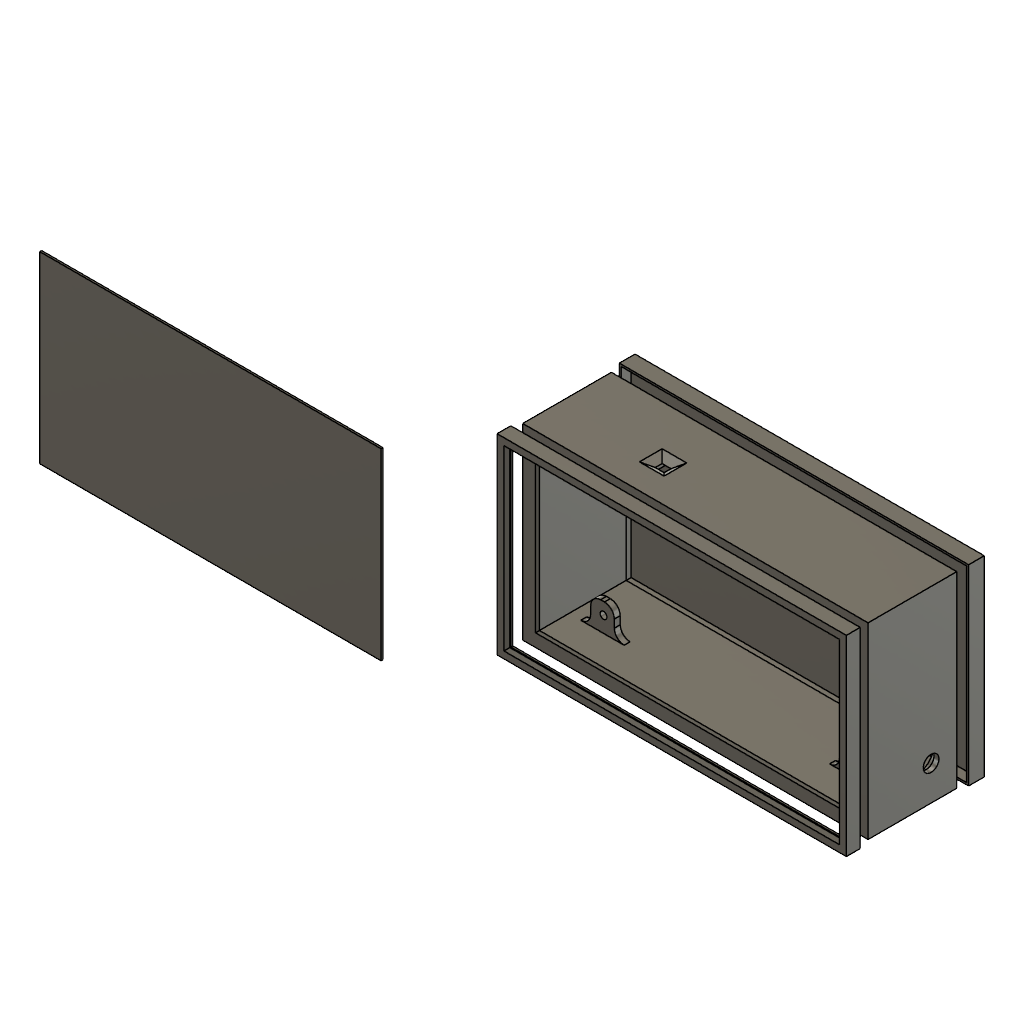
Bedroom Clock (Autodesk Fusion 360 design; units mm, degrees)
Autodesk Fusion 360 part; units mm, degrees
sketch "Sketch1" plane through (0, 0, 0) normal (0, 0, 1) x (1, 0, 0)
  line L0 (80.1, -40.1) -> (-80.1, -40.1)
  line L1 (-80.1, -40.1) -> (-80.1, 40.1)
  line L2 (-80.1, 40.1) -> (80.1, 40.1)
  line L3 (80.1, 40.1) -> (80.1, -40.1)
  line L4 (80.1, -40.1) -> (-80.1, 40.1) construction
  line L5 (-80.1, -40.1) -> (80.1, 40.1) construction
  line L6 (87.6, -47.6) -> (-87.6, -47.6)
  line L7 (-87.6, -47.6) -> (-87.6, 47.6)
  line L8 (-87.6, 47.6) -> (87.6, 47.6)
  line L9 (87.6, 47.6) -> (87.6, -47.6)
  dimension "d1" = 160.2
  dimension "d2" = 80.2
  dimension "d3" = -7.5
  constraint horizontal L0
  constraint perpendicular L0 L1
  constraint parallel L0 L2
  constraint parallel L1 L3
  constraint coincident L4 origin
  constraint coincident L5 origin
  measures "d1" distance of L1.end L2.end
  measures "d2" distance of L0.end L1.end
extrude "Extrude1" add sketch "Sketch1" along normal blind 30 makes body 1
sketch "Sketch2" plane through (0, -40.1, 0) normal (0, 1, 0) x (-1, 0, 0)
  line L0 (-80.1, 0) -> (80.1, 0)
  line L1 (80.1, 0) -> (80.1, 30)
  line L2 (80.1, 30) -> (-80.1, 30)
  line L3 (-80.1, 30) -> (-80.1, 0)
  line L4 (69.1, 11) -> (57.1, 11)
  line L5 (57.1, 11) -> (57.1, 14)
  line L6 (57.1, 14) -> (69.1, 14)
  line L7 (69.1, 14) -> (69.1, 11)
  line L8 (-57.1, 11) -> (-69.1, 11)
  line L9 (-69.1, 11) -> (-69.1, 14)
  line L10 (-69.1, 14) -> (-57.1, 14)
  line L11 (-57.1, 14) -> (-57.1, 11)
  dimension "d6" = 12
  dimension "d7" = 11
  dimension "d8" = 16
  dimension "d9" = 12
  dimension "d10" = 3
  dimension "d11" = 16
  dimension "d12" = 11
  constraint horizontal L4
  constraint vertical L5
  constraint horizontal L6
  constraint vertical L7
  constraint horizontal L8
  constraint vertical L9
  constraint horizontal L10
  constraint vertical L11
  measures "d6" distance of L4.start L4.end
  measures "d7" distance of L1 L7
  measures "d8" distance of L2 L6
  measures "d9" distance of L8.start L8.end
  measures "d10" distance of L8.start L10.end
  measures "d11" distance of L2 L10
  measures "d12" distance of L3 L9
extrude "Extrude2" add sketch "Sketch2" along normal blind 14 contours L4 L5 L6 L7 | L8 L9 L10 L11 bodies 1
mirror "Mirror1" about plane through (0, 0, 0) normal (0, 1, 0) of "Extrude2"
fillet "Fillet2" radius 5 16 edges at (-57.1, -40.1, 12.5) (-57.1, -26.1, 12.5) (-69.1, -26.1, 12.5) (-69.1, -40.1, 12.5) (57.1, -40.1, 12.5) (57.1, -26.1, 12.5) (69.1, -26.1, 12.5) (69.1, -40.1, 12.5) (-57.1, 40.1, 12.5) (-57.1, 26.1, 12.5) (-69.1, 26.1, 12.5) (-69.1, 40.1, 12.5) (57.1, 40.1, 12.5) (57.1, 26.1, 12.5) (69.1, 26.1, 12.5) (69.1, 40.1, 12.5) on bodies 1
sketch "Sketch4" plane through (0, 0, 14) normal (0, 0, 1) x (1, 0, 0)
  arc A0 (-64.1, -26.1) -> (-69.1, -31.1) centre (-64.1, -31.1) ccw
  line L0 (-69.1, -31.1) -> (-69.1, -35.1)
  arc A1 (-74.1, -40.1) -> (-69.1, -35.1) centre (-74.1, -35.1) ccw
  line L1 (-74.1, -40.1) -> (-52.1, -40.1)
  arc A2 (-57.1, -35.1) -> (-52.1, -40.1) centre (-52.1, -35.1) ccw
  line L2 (-57.1, -35.1) -> (-57.1, -31.1)
  arc A3 (-57.1, -31.1) -> (-62.1, -26.1) centre (-62.1, -31.1) ccw
  line L3 (-62.1, -26.1) -> (-64.1, -26.1)
  circle A4 centre (-62.57, -32.17) radius 1.75
  line L4 (-74.1, -40.1) -> (-52.1, -40.1)
  circle A5 centre (62.57, -32.17) radius 1.75
  line L5 (74.1, -40.1) -> (52.1, -40.1)
  circle A6 centre (62.57, 32.17) radius 1.75
  line L6 (52.1, 40.1) -> (74.1, 40.1)
  circle A7 centre (-62.57, 32.17) radius 1.75
  line L7 (-74.1, 40.1) -> (-52.1, 40.1)
  point P0 (-80.1, -40.1)
  point P1 (80.1, -40.1)
  point P2 (80.1, 40.1)
  point P3 (-80.1, 40.1)
  dimension "d28" = 3.5
  dimension "d29" = 7.93
  dimension "d30" = 17.53
  dimension "d31" = 3.5
  dimension "d32" = 7.93
  dimension "d33" = 17.53
  dimension "d34" = 3.5
  dimension "d35" = 7.93
  dimension "d36" = 17.53
  dimension "d37" = 3.5
  dimension "d38" = 7.93
  dimension "d39" = 17.53
  measures "d28" diameter of A4
  measures "d29" distance of A4.centre L4
  measures "d30" horizontal distance of A4.centre P0
  measures "d31" diameter of A5
  measures "d32" distance of A5.centre L5
  measures "d33" horizontal distance of A5.centre P1
  measures "d34" diameter of A6
  measures "d35" distance of A6.centre L6
  measures "d36" horizontal distance of A6.centre P2
  measures "d37" diameter of A7
  measures "d38" distance of A7.centre L7
  measures "d39" horizontal distance of A7.centre P3
extrude "Extrude4" cut sketch "Sketch4" against normal blind 3 contours A4 | A5 | A6 | A7 bodies 1
chamfer "Chamfer1" distance 1 angle 45 4 edges at (-80.1, 0, 30) (0, -40.1, 30) (0, 40.1, 30) (80.1, 0, 30) tangent chain off on bodies 1
ref_plane "WorkPlane1" through (0, 0, 10) normal (0, 0, 1) x (1, 0, 0) in component "ESP32 Mount"
sketch "Sketch1 (2)" plane through (0, 0, 10) normal (0, 0, 1) x (1, 0, 0) in component "ESP32 Mount"
  line L0 (62, -36.7675) -> (-62, -36.7675)
  line L1 (-70, -28.7675) -> (-70, 28.7675)
  line L2 (-62, 36.7675) -> (62, 36.7675)
  line L3 (70, 28.7675) -> (70, -28.7675)
  line L4 (5, -9.7675) -> (-14, -9.7675)
  line L5 (-14, -9.7675) -> (-14, 10.2325)
  line L6 (-14, 10.2325) -> (5, 10.2325)
  line L7 (5, 10.2325) -> (5, -9.7675)
  circle A0 centre (-62.57, 32.17) radius 1.75
  circle A1 centre (-62.57, -32.17) radius 1.75
  circle A2 centre (62.57, -32.17) radius 1.75
  circle A3 centre (62.57, 32.17) radius 1.75
  line L8 (-46.57, 15.83) -> (-31.57, 15.83)
  line L9 (-31.57, 15.83) -> (-31.57, -17.17)
  line L10 (-31.57, -17.17) -> (-46.57, -17.17)
  line L11 (-46.57, -17.17) -> (-46.57, 15.83)
  circle A4 centre (18.7, 12.17) radius 1.5
  circle A5 centre (59, 12.17) radius 1.5
  circle A6 centre (18.7, -7.13) radius 1.5
  circle A7 centre (59, -7.13) radius 1.5
  arc A8 (-62, 36.7675) -> (-70, 28.7675) centre (-62, 28.7675) ccw
  arc A9 (-70, -28.7675) -> (-62, -36.7675) centre (-62, -28.7675) ccw
  arc A10 (62, -36.7675) -> (70, -28.7675) centre (62, -28.7675) ccw
  arc A11 (70, 28.7675) -> (62, 36.7675) centre (62, 28.7675) ccw
  dimension "d45" = 65
  dimension "d46" = 27
  dimension "d48" = 15
  dimension "d49" = 33
  dimension "d50" = 15
  dimension "d51" = 16
  dimension "d52" = 3
  dimension "d53" = 3
  dimension "d54" = 3
  dimension "d55" = 3
  dimension "d56" = 19.3
  dimension "d57" = 19.3
  dimension "d58" = 40.3
  dimension "d59" = 40.3
  dimension "d60" = 11
  dimension "d61" = 11
  dimension "d62" = 20
  dimension "d63" = 20
  dimension "d64" = 8
  dimension "d67" = 19
  dimension "d68" = 140
  dimension "d69" = 20
  constraint horizontal L0
  constraint perpendicular L0 L1
  constraint parallel L0 L2
  constraint parallel L1 L3
  constraint horizontal L4
  constraint perpendicular L4 L5
  constraint parallel L4 L6
  constraint parallel L5 L7
  constraint horizontal L8
  constraint vertical L9
  constraint horizontal L10
  constraint vertical L11
  constraint tangent L2 A8
  constraint tangent L1 A8
  constraint tangent L0 A9
  constraint tangent L1 A9
  constraint equal A8 A9
  constraint tangent L0 A10
  constraint tangent L3 A10
  constraint equal A8 A10
  constraint tangent L3 A11
  constraint tangent L2 A11
  constraint equal A8 A11
  measures "d45" distance of L3 L7
  measures "d46" distance of L0 L4
  measures "d48" distance of L8.start L8.end
  measures "d49" distance of L8.start L10.end
  measures "d50" distance of A1.centre L10
  measures "d51" distance of A0.centre L11
  measures "d52" diameter of A4
  measures "d53" diameter of A5
  measures "d54" diameter of A6
  measures "d55" diameter of A7
  measures "d56" vertical distance of A5.centre A7.centre
  measures "d57" vertical distance of A4.centre A6.centre
  measures "d58" horizontal distance of A6.centre A7.centre
  measures "d59" horizontal distance of A4.centre A5.centre
  measures "d60" distance of L3 A7.centre
  measures "d61" distance of L3 A5.centre
  measures "d62" vertical distance of A3.centre A5.centre
  measures "d63" vertical distance of A3.centre A4.centre
  measures "d64" radius of A8
  measures "d67" distance of L5 L7
  measures "d68" distance of L1 L3
  measures "d69" distance of L4 L6
extrude "Extrude1'" add sketch "Sketch1 (2)" along normal blind 3 separate body makes body 2 in component "ESP32 Mount"
move_body "Move1" bodies 2 to x (1, 0, 0) y (0, 1, 0) z (0, 0, 1) at (0, 0, 65) in component "ESP32 Mount"
copy_body "Body->Comp1" bodies 1 removing the originals makes body 3 in component "Display Frame"
sketch "Sketch1 (3)" plane through (0, 40.1, 0) normal (0, -1, 0) x (1, 0, 0) in component "Display Frame"
  line L0 (80.1, 29) -> (-80.1, 29)
  line L1 (-80.1, 29) -> (-80.1, 0)
  line L2 (-80.1, 0) -> (80.1, 0)
  line L3 (80.1, 0) -> (80.1, 29)
  line L4 (74.1, 11) -> (52.1, 11)
  line L5 (52.1, 11) -> (52.1, 14)
  line L6 (52.1, 14) -> (74.1, 14)
  line L7 (74.1, 14) -> (74.1, 11)
  line L8 (-74.1, 14) -> (-52.1, 14)
  line L9 (-52.1, 14) -> (-52.1, 11)
  line L10 (-52.1, 11) -> (-74.1, 11)
  line L11 (-74.1, 11) -> (-74.1, 14)
  line L12 (-28.5, 0) -> (-42.1, 0)
  line L13 (-42.1, 0) -> (-42.1, 18.5)
  line L14 (-42.1, 18.5) -> (-28.5, 18.5)
  line L15 (-28.5, 18.5) -> (-28.5, 0)
  line L16 (-32.6, 9.75) -> (-37.1, 9.75)
  line L17 (-37.1, 9.75) -> (-37.1, 13.25)
  line L18 (-37.1, 13.25) -> (-32.6, 13.25)
  line L19 (-32.6, 13.25) -> (-32.6, 9.75)
  dimension "d70" = 38
  dimension "d71" = 13.6
  dimension "d72" = 18.5
  dimension "d73" = 4.5
  dimension "d74" = 3.5
  dimension "d75" = 5
  dimension "d76" = 5.25
  constraint horizontal L12
  constraint vertical L13
  constraint horizontal L14
  constraint vertical L15
  constraint coincident L2 L12.start
  constraint horizontal L16
  constraint vertical L17
  constraint horizontal L18
  constraint vertical L19
  measures "d70" distance of L1 L13
  measures "d71" distance of L13 L15
  measures "d72" distance of L12 L14
  measures "d73" distance of L16.start L16.end
  measures "d74" distance of L16.start L18.end
  measures "d75" distance of L13 L17
  measures "d76" distance of L14 L18
extrude "Extrude1''" cut sketch "Sketch1 (3)" against normal blind 5 contours L2 L12 L13 L14 L15 bodies 3 in component "Display Frame"
extrude "Extrude2'" cut 1 faces at (-34.1, 40.1, 12.0833) along direction (0, 1, 0) blind 7.5 on bodies 3 bodies 3 in component "Display Frame"
chamfer "Chamfer1'" distance 4 distance2 2.5 4 edges at (-34.85, 47.6, 13.25) (-32.6, 47.6, 11.5) (-34.85, 47.6, 9.75) (-37.1, 47.6, 11.5) measured on face at (47.5333, 47.6, 14.4167) measured on face at (47.5333, 47.6, 14.4167) measured on face at (47.5333, 47.6, 14.4167) measured on face at (47.5333, 47.6, 14.4167) tangent chain off on bodies 3 in component "Display Frame"
sketch "Sketch2 (2)" plane through (-28.5, 0, 0) normal (-1, 0, 0) x (0, 0, 1) in component "Display Frame"
  line L0 (0, 40.1) -> (18.5, 40.1)
  line L1 (18.5, 40.1) -> (18.5, 45.1)
  line L2 (18.5, 45.1) -> (0, 45.1)
  line L3 (0, 45.1) -> (0, 40.1)
  line L4 (18.5, 42.5) -> (4, 42.5)
  line L5 (4, 42.5) -> (4, 40.5)
  line L6 (4, 40.5) -> (18.5, 40.5)
  line L7 (18.5, 40.5) -> (18.5, 42.5)
  dimension "d82" = 14.5
  dimension "d83" = 2
  dimension "d84" = 2.6
  constraint horizontal L4
  constraint vertical L5
  constraint horizontal L6
  constraint vertical L7
  measures "d82" distance of L4.start L4.end
  measures "d83" distance of L4.start L6.end
  measures "d84" distance of L2 L4
extrude "Extrude3" add sketch "Sketch2 (2)" along normal blind 2 contours L1 L4 L5 L6 L7 bodies 3 in component "Display Frame"
chamfer "Chamfer2" distance 2 distance2 1 1 edges at (-29.5, 42.5, 4) measured on face at (-29.1667, 42.5, 13.6667) tangent chain off on bodies 3 in component "Display Frame"
sketch "Sketch3" plane through (-42.1, 0, 0) normal (1, 0, 0) x (0, 0, -1) in component "Display Frame"
  line L0 (-18.5, 40.1) -> (0, 40.1)
  line L1 (0, 40.1) -> (0, 45.1)
  line L2 (0, 45.1) -> (-18.5, 45.1)
  line L3 (-18.5, 45.1) -> (-18.5, 40.1)
  line L4 (-18.5, 42.5) -> (-4, 42.5)
  line L5 (-4, 42.5) -> (-4, 40.5)
  line L6 (-4, 40.5) -> (-18.5, 40.5)
  line L7 (-18.5, 40.5) -> (-18.5, 42.5)
  dimension "d89" = 14.5
  dimension "d90" = 2
  dimension "d91" = 2.6
  constraint horizontal L4
  constraint vertical L5
  constraint horizontal L6
  constraint vertical L7
  constraint coincident L3 L4.start
  measures "d89" distance of L4.start L4.end
  measures "d90" distance of L4.start L6.end
  measures "d91" distance of L2 L4
extrude "Extrude4'" add sketch "Sketch3" along normal blind 2 contours L3 L4 L5 L6 L7 bodies 3 in component "Display Frame"
chamfer "Chamfer3" distance 1 distance2 2 1 edges at (-41.1, 42.5, 4) measured on face at (-41.4333, 41.8333, 4) tangent chain off on bodies 3 in component "Display Frame"
sketch "Sketch1 (4)" plane through (0, 0, 0) normal (0, 0, 1) x (1, 0, 0) in component "Film Template"
  line L0 (87.6, 47.6) -> (-87.6, 47.6)
  line L1 (-87.6, 47.6) -> (-87.6, -47.6)
  line L2 (-87.6, -47.6) -> (87.6, -47.6)
  line L3 (87.6, -47.6) -> (87.6, 47.6)
  line L4 (-86.6, -46.6) -> (86.6, -46.6)
  line L5 (86.6, -46.6) -> (86.6, 46.6)
  line L6 (86.6, 46.6) -> (-86.6, 46.6)
  line L7 (-86.6, 46.6) -> (-86.6, -46.6)
  dimension "d97" = -1
extrude "Extrude1'''" add sketch "Sketch1 (4)" along normal blind 1 separate body contours L4 L5 L6 L7 makes body 4 in component "Film Template"
move_body "Move1'" bodies 4 to x (1, 0, 0) y (0, 1, 0) z (0, 0, 1) at (0, 0, 75) in component "Film Template"
extrude "Extrude5" add 1 faces at (-26.7, -45.1, 0) along direction (0, 0, -1) blind 15 on bodies 3 bodies 3 in component "Display Frame"
sketch "Sketch4 (2)" plane through (80.1, 0, 0) normal (-1, 0, 0) x (0, 0, 1) in component "Display Frame"
  line L0 (29, -40.1) -> (29, 40.1)
  line L1 (29, 40.1) -> (-15, 40.1)
  line L2 (-15, 40.1) -> (-15, -40.1)
  line L3 (-15, -40.1) -> (29, -40.1)
  circle A0 centre (-2, -30.1) radius 9
  circle A1 centre (-2, -30.1) radius 4
  dimension "d102" = 18
  dimension "d103" = 10
  dimension "d104" = 13
  dimension "d105" = 8
  constraint concentric A0 A1
  measures "d102" diameter of A0
  measures "d103" distance of L3 A0.centre
  measures "d104" distance of L2 A0.centre
  measures "d105" diameter of A1
extrude "Extrude6" cut sketch "Sketch4 (2)" against normal blind 5 contours A0 bodies 3 in component "Display Frame"
extrude "Extrude7" cut 1 faces at (80.1, -31.2547, -2.6667) along direction (1, 0, 0) blind 7.5 on bodies 3 bodies 3 in component "Display Frame"
ref_plane "WorkPlane1" through (0, 0, 35) normal (0, 0, 1) x (1, 0, 0) in component "Film Holder"
sketch "Sketch1 (5)" plane through (0, 0, 35) normal (0, 0, 1) x (1, 0, 0) in component "Film Holder"
  line L0 (87.6, 47.6) -> (-87.6, 47.6)
  line L1 (-87.6, 47.6) -> (-87.6, -47.6)
  line L2 (-87.6, -47.6) -> (87.6, -47.6)
  line L3 (87.6, -47.6) -> (87.6, 47.6)
  line L4 (-87.6, -47.6) -> (87.6, -47.6)
  line L5 (87.6, -47.6) -> (87.6, 47.6)
  line L6 (87.6, 47.6) -> (-87.6, 47.6)
  line L7 (-87.6, 47.6) -> (-87.6, -47.6)
  line L8 (-88.6, -48.6) -> (88.6, -48.6)
  line L9 (88.6, -48.6) -> (88.6, 48.6)
  line L10 (88.6, 48.6) -> (-88.6, 48.6)
  line L11 (-88.6, 48.6) -> (-88.6, -48.6)
  line L12 (-83.6, -43.6) -> (83.6, -43.6)
  line L13 (83.6, -43.6) -> (83.6, 43.6)
  line L14 (83.6, 43.6) -> (-83.6, 43.6)
  line L15 (-83.6, 43.6) -> (-83.6, -43.6)
  dimension "d112" = 0
  dimension "d113" = 1
  dimension "d114" = -4
  measures "d112" distance of L0
extrude "Extrude1''''" add sketch "Sketch1 (5)" along normal blind 2 separate body contours L0 L1 L2 L3 L4 L5 L6 L7 | L8 L9 L10 L11 makes body 5 in component "Film Holder"
extrude "Extrude2''" add sketch "Sketch1 (5)" against normal blind 5 contours L8 L9 L10 L11 bodies 5 in component "Film Holder"
chamfer "Chamfer1''" distance 1.5 angle 45 4 edges at (0, 43.6, 37) (-83.6, 0, 37) (0, -43.6, 37) (83.6, 0, 37) tangent chain off on bodies 5 in component "Film Holder"
ref_plane "WorkPlane1" through (0, 0, -20) normal (0, 0, 1) x (1, 0, 0) in component "Back"
sketch "Sketch1 (6)" plane through (0, 0, -20) normal (0, 0, 1) x (1, 0, 0) in component "Back"
  line L0 (87.6, -47.6) -> (-87.6, -47.6)
  line L1 (-87.6, -47.6) -> (-87.6, 47.6)
  line L2 (-87.6, 47.6) -> (87.6, 47.6)
  line L3 (87.6, 47.6) -> (87.6, -47.6)
  line L4 (87.6, -47.6) -> (-87.6, -47.6)
  line L5 (-87.6, -47.6) -> (-87.6, 47.6)
  line L6 (-87.6, 47.6) -> (87.6, 47.6)
  line L7 (87.6, 47.6) -> (87.6, -47.6)
  line L8 (88.6, -48.6) -> (-88.6, -48.6)
  line L9 (-88.6, -48.6) -> (-88.6, 48.6)
  line L10 (-88.6, 48.6) -> (88.6, 48.6)
  line L11 (88.6, 48.6) -> (88.6, -48.6)
  dimension "d122" = 0
  dimension "d123" = -1
  measures "d122" distance of L2
extrude "Extrude1'''''" add sketch "Sketch1 (6)" against normal blind 3 separate body contours L0 L1 L2 L3 L4 L5 L6 L7 | L8 L9 L10 L11 makes body 6 in component "Back"
extrude "Extrude2'''" add sketch "Sketch1 (6)" along normal blind 5 bodies 6 in component "Back"
component "ESP32 Mount" placed x (1, 0, 0) y (0, 1, 0) z (0, 0, 1) at (0, 0, 0)
component "Display Frame" placed x (1, 0, 0) y (0, 1, 0) z (0, 0, 1) at (0, 0, 0)
component "Film Template" placed x (1, 0, 0) y (0, 1, 0) z (0, 0, 1) at (0, 0, 0)
component "Film Holder" placed x (1, 0, 0) y (0, 1, 0) z (0, 0, 1) at (0, 0, 0)
component "Back" placed x (1, 0, 0) y (0, 1, 0) z (0, 0, 1) at (0, 0, 0)
component "Bedroom Clock v8" placed x (1, 0, 0) y (0, 1, 0) z (0, 0, 1) at (0, 0, 0) in component "Film Holder"
